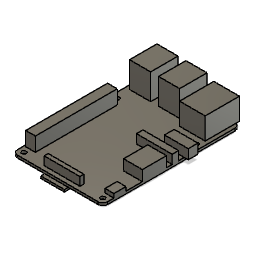
tut_v3.f3d v1 (Autodesk Fusion 360 archive; units mm, degrees)
design "Rough Pi Model"
Autodesk Fusion 360 part; units mm, degrees
sketch "PCB" plane through (0, 0, 0) normal (0, 1, 0) x (1, 0, 0) in component "Raspberry Pi Master"
  line L0 (3, 0) -> (53, 0)
  line L1 (56, -3) -> (56, -82)
  line L2 (53, -85) -> (3, -85)
  line L3 (0, -82) -> (0, -3)
  arc A0 (3, 0) -> (0, -3) centre (3, -3) ccw
  arc A1 (56, -3) -> (53, 0) centre (53, -3) ccw
  arc A2 (53, -85) -> (56, -82) centre (53, -82) ccw
  arc A3 (0, -82) -> (3, -85) centre (3, -82) ccw
  circle A4 centre (52.5, -81.5) radius 1.375
  circle A5 centre (3.5, -81.5) radius 1.375
  circle A6 centre (3.5, -23.5) radius 1.375
  line L4 (3.5, -81.5) -> (3.5, -23.5) construction
  circle A7 centre (52.5, -23.5) radius 1.375
  line L5 (52.5, -23.5) -> (3.5, -23.5) construction
  line L6 (52.5, -23.5) -> (52.5, -81.5) construction
  point P0 (56, 0)
  point P1 (0, -85)
  dimension "d1" = 56
  dimension "d2" = 85
  dimension "d3" = 3
  dimension "d4" = 3
  dimension "d5" = 3
  dimension "d6" = 3
  dimension "d7" = 2.75
  dimension "d8" = 3.5
  dimension "d9" = 3.5
  dimension "d10" = 3.5
  dimension "d11" = 3.5
  dimension "d12" = 58
  constraint horizontal L0
  constraint vertical L1
  constraint horizontal L2
  constraint vertical L3
  constraint coincident origin L3
  constraint coincident origin L0
  constraint tangent L3 A0
  constraint tangent L0 A0
  constraint coincident P0 L0
  constraint coincident P0 L1
  constraint tangent L0 A1
  constraint tangent L1 A1
  constraint tangent L1 A2
  constraint tangent L2 A2
  constraint coincident P1 L2
  constraint coincident P1 L3
  constraint tangent L2 A3
  constraint tangent L3 A3
  constraint equal A4 A5
  constraint coincident A5.centre L4.start
  constraint coincident A6.centre L4.end
  constraint vertical L4
  constraint coincident A7.centre L5.start
  constraint coincident A4.centre L6.end
  constraint vertical L6
  constraint horizontal L5
  constraint equal A4 A7
  constraint equal A4 A6
  measures "d1" distance of origin P0
  measures "d2" distance of origin P1
  measures "d3" radius of A0
  measures "d4" radius of A1
  measures "d5" radius of A2
  measures "d6" radius of A3
  measures "d7" diameter of A4
  measures "d8" distance of L2 A4.centre
  measures "d9" distance of L1 A4.centre
  measures "d10" distance of L2 A5.centre
  measures "d11" distance of L3 A5.centre
  measures "d12" vertical distance of A5.centre A6.centre
extrude "Extrude1" add sketch "PCB" along normal blind 1.5 in component "Raspberry Pi Master"
sketch "Front IO" plane through (0, 1.5, 0) normal (0, 1, 0) x (-1, 0, 0) in component "Raspberry Pi Master"
  circle A0 centre (-52.5, 81.5) radius 1.375
  circle A1 centre (-3.5, 81.5) radius 1.375
  circle A2 centre (-3.5, 23.5) radius 1.375
  circle A3 centre (-52.5, 23.5) radius 1.375
  arc A4 (-3, 0) -> (0, 3) centre (-3, 3) ccw
  line L0 (0, 3) -> (0, 82)
  arc A5 (0, 82) -> (-3, 85) centre (-3, 82) ccw
  line L1 (-3, 85) -> (-53, 85)
  arc A6 (-53, 85) -> (-56, 82) centre (-53, 82) ccw
  line L2 (-56, 82) -> (-56, 3)
  arc A7 (-56, 3) -> (-53, 0) centre (-53, 3) ccw
  line L3 (-53, 0) -> (-3, 0)
  line L4 (-2.45, -2.1) -> (-15.55, -2.1)
  line L5 (-15.55, -2.1) -> (-15.55, 14.9)
  line L6 (-15.55, 14.9) -> (-2.45, 14.9)
  line L7 (-2.45, 14.9) -> (-2.45, -2.1)
  line L8 (-20.45, -2.1) -> (-33.55, -2.1)
  line L9 (-33.55, -2.1) -> (-33.55, 14.9)
  line L10 (-33.55, 14.9) -> (-20.45, 14.9)
  line L11 (-20.45, 14.9) -> (-20.45, -2.1)
  line L12 (-27, -2.1) -> (-56, -2.1) construction
  line L13 (-9, -2.1) -> (-27, -2.1) construction
  line L14 (-56, 3) -> (-56, -2.1) construction
  line L15 (-53.65, -2.1) -> (-37.75, -2.1)
  line L16 (-37.75, -2.1) -> (-37.75, 19.15)
  line L17 (-37.75, 19.15) -> (-53.65, 19.15)
  line L18 (-53.65, 19.15) -> (-53.65, -2.1)
  line L19 (-15.55, 14.9) -> (-20.45, 14.9) construction
  dimension "d15" = 29
  dimension "d16" = 47
  dimension "d17" = 13.1
  dimension "d18" = 2.1
  dimension "d19" = 4.2
  dimension "d21" = 15.9
  dimension "d22" = 21.25
  dimension "d23" = 17
  constraint horizontal L4
  constraint vertical L5
  constraint horizontal L6
  constraint vertical L7
  constraint horizontal L8
  constraint vertical L9
  constraint horizontal L10
  constraint vertical L11
  constraint midpoint L8 L12.start
  constraint parallel L8 L12
  constraint midpoint L4 L13.start
  constraint parallel L4 L13
  constraint coincident L2.end A7.start
  constraint tangent A7 L14
  constraint coincident L12.end L14.end
  constraint equal L6 L10
  constraint horizontal L15
  constraint vertical L16
  constraint horizontal L17
  constraint vertical L18
  constraint coincident L12 L15.start
  constraint horizontal L19
  measures "d15" distance of L12.start L12.end
  measures "d16" distance of L12.end L13.start
  measures "d17" distance of L9.end L10.end
  measures "d18" distance of L3 L12
  measures "d19" distance of L9 L16
  measures "d21" distance of L16.end L17.end
  measures "d22" distance of L15.start L17.end
  measures "d23" distance of L8 L10
extrude "Extrude2" add sketch "Front IO" along normal blind 13.5 contours A7 L3 L15 L16 L18 | A7 L3 L16 L17 L18 in component "Raspberry Pi Master"
extrude "Extrude3" add sketch "Front IO" along normal blind 16 contours A4 L3 L5 L6 L7 | A4 L3 L4 L5 L7 | L3 L8 L9 L11 | L3 L9 L10 L11 in component "Raspberry Pi Master"
sketch "Right IO" plane through (0, 1.5, 0) normal (0, 1, 0) x (-1, 0, 0) in component "Raspberry Pi Master"
  line L0 (-20.45, 14.9) -> (-20.45, 0)
  line L1 (-20.45, 0) -> (-15.55, 0)
  line L2 (-15.55, 0) -> (-15.55, 14.9)
  line L3 (-15.55, 14.9) -> (-2.45, 14.9)
  line L4 (-2.45, 14.9) -> (-2.45, 0.0508)
  arc A0 (-2.45, 0.0508) -> (0, 3) centre (-3, 3) ccw
  line L5 (0, 3) -> (0, 82)
  arc A1 (0, 82) -> (-3, 85) centre (-3, 82) ccw
  line L6 (-3, 85) -> (-53, 85)
  arc A2 (-53, 85) -> (-56, 82) centre (-53, 82) ccw
  line L7 (-56, 82) -> (-56, 3)
  arc A3 (-56, 3) -> (-53.65, 0.0713) centre (-53, 3) ccw
  line L8 (-53.65, 0.0713) -> (-53.65, 19.15)
  line L9 (-53.65, 19.15) -> (-37.75, 19.15)
  line L10 (-37.75, 19.15) -> (-37.75, 0)
  line L11 (-37.75, 0) -> (-33.55, 0)
  line L12 (-33.55, 0) -> (-33.55, 14.9)
  line L13 (-33.55, 14.9) -> (-20.45, 14.9)
  circle A4 centre (-52.5, 81.5) radius 1.375
  circle A5 centre (-3.5, 81.5) radius 1.375
  circle A6 centre (-3.5, 23.5) radius 1.375
  circle A7 centre (-52.5, 23.5) radius 1.375
  line L14 (-50.5, 78.15) -> (-56.1, 78.15)
  line L15 (-56.1, 78.15) -> (-56.1, 70.65)
  line L16 (-56.1, 70.65) -> (-50.5, 70.65)
  line L17 (-50.5, 70.65) -> (-50.5, 78.15)
  line L18 (-44.35, 45.5) -> (-56.1, 45.5)
  line L19 (-56.1, 45.5) -> (-56.1, 60.5)
  line L20 (-56.1, 60.5) -> (-44.35, 60.5)
  line L21 (-44.35, 60.5) -> (-44.35, 45.5)
  line L22 (-56.1, 53) -> (-56.1, 74.4) construction
  line L23 (-56, 42) -> (-33.85, 42)
  line L24 (-33.85, 42) -> (-33.85, 38)
  line L25 (-33.85, 38) -> (-56, 38)
  line L26 (-56, 38) -> (-56, 42)
  line L27 (-58.5, 34.5) -> (-43.75, 34.5)
  line L28 (-43.75, 34.5) -> (-43.75, 28.5)
  line L29 (-43.75, 28.5) -> (-58.5, 28.5)
  line L30 (-58.5, 28.5) -> (-58.5, 34.5)
  point P0 (-56, 40)
  point P1 (-58.5, 31.5)
  dimension "d28" = 10.6
  dimension "d29" = 32
  dimension "d30" = 13
  dimension "d31" = 53.5
  dimension "d32" = 7.5
  dimension "d33" = 15
  dimension "d34" = 4
  dimension "d35" = 6
  dimension "d36" = 58.5
  dimension "d37" = 5.6
  dimension "d38" = 0.1
  dimension "d39" = 11.75
  dimension "d40" = 22.15
  dimension "d41" = 14.75
  constraint horizontal L14
  constraint vertical L15
  constraint horizontal L16
  constraint vertical L17
  constraint horizontal L18
  constraint vertical L19
  constraint horizontal L20
  constraint vertical L21
  constraint midpoint L19 L22.start
  constraint midpoint L15 L22.end
  constraint vertical L22
  constraint horizontal L23
  constraint vertical L24
  constraint horizontal L25
  constraint vertical L26
  constraint coincident L7 L23.start
  constraint midpoint L26 P0
  constraint horizontal L27
  constraint vertical L28
  constraint horizontal L29
  constraint vertical L30
  constraint midpoint L30 P1
  measures "d28" distance of L6 L22.end
  measures "d29" distance of L6 L22.start
  measures "d30" vertical distance of L22.start P0
  measures "d31" distance of L6 P1
  measures "d32" distance of L14.start L16.end
  measures "d33" distance of L18.start L20.end
  measures "d34" distance of L23.end L24.end
  measures "d35" distance of L27.end L28.end
  measures "d36" distance of L5 L30
  measures "d37" distance of L15 L17
  measures "d38" distance of L7 L22
  measures "d39" distance of L19 L21
  measures "d40" distance of L24 L26
  measures "d41" distance of L28 L30
extrude "Extrude4" add sketch "Right IO" along normal blind 6 contours L7 L27 L29 L30 | L7 L27 L28 L29 in component "Raspberry Pi Master"
extrude "Extrude5" add sketch "Right IO" along normal blind 5.5 contours L7 L23 L24 L25 L26 in component "Raspberry Pi Master"
extrude "Extrude6" add sketch "Right IO" along normal blind 6.5 contours L7 L18 L20 L21 in component "Raspberry Pi Master"
extrude "Extrude7" add sketch "Right IO" along normal blind 2.45 contours L7 L14 L16 L17 in component "Raspberry Pi Master"
sketch "SD Card" plane through (0, 0, 0) normal (0, -1, 0) x (1, 0, 0) in component "Raspberry Pi Master"
  circle A0 centre (52.5, 81.5) radius 1.375
  circle A1 centre (3.5, 81.5) radius 1.375
  circle A2 centre (3.5, 23.5) radius 1.375
  circle A3 centre (52.5, 23.5) radius 1.375
  arc A4 (0, 3) -> (3, 0) centre (3, 3) ccw
  line L0 (3, 0) -> (53, 0)
  arc A5 (53, 0) -> (56, 3) centre (53, 3) ccw
  line L1 (56, 3) -> (56, 82)
  arc A6 (56, 82) -> (53, 85) centre (53, 82) ccw
  line L2 (53, 85) -> (3, 85)
  arc A7 (3, 85) -> (0, 82) centre (3, 82) ccw
  line L3 (0, 82) -> (0, 3)
  line L4 (34.5, 87.42) -> (19.9, 87.42)
  line L5 (19.9, 87.42) -> (19.9, 70.4)
  line L6 (19.9, 70.4) -> (34.5, 70.4)
  line L7 (34.5, 70.4) -> (34.5, 87.42)
  dimension "d51" = 19.9
  dimension "d52" = 14.6
  dimension "d53" = 14.6
  dimension "d54" = 2.42
  constraint horizontal L4
  constraint vertical L5
  constraint horizontal L6
  constraint vertical L7
  measures "d51" distance of L3 L5
  measures "d52" distance of L4.start L4.end
  measures "d53" distance of L2 L6
  measures "d54" distance of L2 L4
extrude "Extrude8" add sketch "SD Card" along normal blind 1.35 contours L2 L4 L5 L7 | L2 L5 L6 L7 in component "Raspberry Pi Master"
sketch "Back IO" plane through (0, 1.5, 0) normal (0, 1, 0) x (-1, 0, 0) in component "Raspberry Pi Master"
  arc A0 (3, 85) -> (0, 82) centre (3, 82) ccw
  circle A1 centre (-52.5, 81.5) radius 1.375
  circle A2 centre (-3.5, 81.5) radius 1.375
  circle A3 centre (-3.5, 23.5) radius 1.375
  circle A4 centre (-52.5, 23.5) radius 1.375
  line L0 (-56, 78.15) -> (-50.5, 78.15)
  line L1 (-50.5, 78.15) -> (-50.5, 70.65)
  line L2 (-50.5, 70.65) -> (-56, 70.65)
  line L3 (-56, 70.65) -> (-56, 60.5)
  line L4 (-56, 60.5) -> (-44.35, 60.5)
  line L5 (-44.35, 60.5) -> (-44.35, 45.5)
  line L6 (-44.35, 45.5) -> (-56, 45.5)
  line L7 (-56, 45.5) -> (-56, 42)
  line L8 (-56, 42) -> (-33.85, 42)
  line L9 (-33.85, 42) -> (-33.85, 38)
  line L10 (-33.85, 38) -> (-56, 38)
  line L11 (-56, 38) -> (-56, 34.5)
  line L12 (-56, 34.5) -> (-43.75, 34.5)
  line L13 (-43.75, 34.5) -> (-43.75, 28.5)
  line L14 (-43.75, 28.5) -> (-56, 28.5)
  line L15 (-56, 28.5) -> (-56, 3)
  arc A5 (-56, 3) -> (-53.65, 0.0713) centre (-53, 3) ccw
  line L16 (-53.65, 0.0713) -> (-53.65, 19.15)
  line L17 (-53.65, 19.15) -> (-37.75, 19.15)
  line L18 (-37.75, 19.15) -> (-37.75, 0)
  line L19 (-37.75, 0) -> (-33.55, 0)
  line L20 (-33.55, 0) -> (-33.55, 14.9)
  line L21 (-33.55, 14.9) -> (-20.45, 14.9)
  line L22 (-20.45, 14.9) -> (-20.45, 0)
  line L23 (-20.45, 0) -> (-15.55, 0)
  line L24 (-15.55, 0) -> (-15.55, 14.9)
  line L25 (-15.55, 14.9) -> (-2.45, 14.9)
  line L26 (-2.45, 14.9) -> (-2.45, 0.0508)
  arc A6 (-2.45, 0.0508) -> (0, 3) centre (-3, 3) ccw
  line L27 (0, 3) -> (0, 82)
  arc A7 (0, 82) -> (-3, 85) centre (-3, 82) ccw
  line L28 (-3, 85) -> (-53, 85)
  arc A8 (-53, 85) -> (-56, 82) centre (-53, 82) ccw
  line L29 (-56, 82) -> (-56, 78.15)
  line L30 (-16.9, 79.85) -> (-39.1, 79.85)
  line L31 (-39.1, 79.85) -> (-39.1, 82.35)
  line L32 (-39.1, 82.35) -> (-16.9, 82.35)
  line L33 (-16.9, 82.35) -> (-16.9, 79.85)
  dimension "d57" = 28
  dimension "d58" = 2.5
  dimension "d59" = 2.65
  dimension "d60" = 22.2
  constraint horizontal L30
  constraint vertical L31
  constraint horizontal L32
  constraint vertical L33
  measures "d58" distance of L30.end L31.end
  measures "d59" distance of L28 L31.end
  measures "d60" distance of L30.start L30.end
extrude "Extrude9" add sketch "Back IO" along normal blind 5.25 contours L30 L31 L32 L33 in component "Raspberry Pi Master"
sketch "GPIO" plane through (0, 1.5, 0) normal (0, 1, 0) x (-1, 0, 0) in component "Raspberry Pi Master"
  arc A0 (-53, 85) -> (-56, 82) centre (-53, 82) ccw
  line L0 (-16.9, 82.35) -> (-16.9, 79.85)
  line L1 (-16.9, 79.85) -> (-39.1, 79.85)
  line L2 (-39.1, 79.85) -> (-39.1, 82.35)
  line L3 (-39.1, 82.35) -> (-16.9, 82.35)
  circle A1 centre (-52.5, 81.5) radius 1.375
  circle A2 centre (-3.5, 81.5) radius 1.375
  circle A3 centre (-3.5, 23.5) radius 1.375
  circle A4 centre (-52.5, 23.5) radius 1.375
  line L4 (-56, 78.15) -> (-50.5, 78.15)
  line L5 (-50.5, 78.15) -> (-50.5, 70.65)
  line L6 (-50.5, 70.65) -> (-56, 70.65)
  line L7 (-56, 70.65) -> (-56, 60.5)
  line L8 (-56, 60.5) -> (-44.35, 60.5)
  line L9 (-44.35, 60.5) -> (-44.35, 45.5)
  line L10 (-44.35, 45.5) -> (-56, 45.5)
  line L11 (-56, 45.5) -> (-56, 42)
  line L12 (-56, 42) -> (-33.85, 42)
  line L13 (-33.85, 42) -> (-33.85, 38)
  line L14 (-33.85, 38) -> (-56, 38)
  line L15 (-56, 38) -> (-56, 34.5)
  line L16 (-56, 34.5) -> (-43.75, 34.5)
  line L17 (-43.75, 34.5) -> (-43.75, 28.5)
  line L18 (-43.75, 28.5) -> (-56, 28.5)
  line L19 (-56, 28.5) -> (-56, 3)
  arc A5 (-56, 3) -> (-53.65, 0.0713) centre (-53, 3) ccw
  line L20 (-53.65, 0.0713) -> (-53.65, 19.15)
  line L21 (-53.65, 19.15) -> (-37.75, 19.15)
  line L22 (-37.75, 19.15) -> (-37.75, 0)
  line L23 (-37.75, 0) -> (-33.55, 0)
  line L24 (-33.55, 0) -> (-33.55, 14.9)
  line L25 (-33.55, 14.9) -> (-20.45, 14.9)
  line L26 (-20.45, 14.9) -> (-20.45, 0)
  line L27 (-20.45, 0) -> (-15.55, 0)
  line L28 (-15.55, 0) -> (-15.55, 14.9)
  line L29 (-15.55, 14.9) -> (-2.45, 14.9)
  line L30 (-2.45, 14.9) -> (-2.45, 0.0508)
  arc A6 (-2.45, 0.0508) -> (0, 3) centre (-3, 3) ccw
  line L31 (0, 3) -> (0, 82)
  arc A7 (0, 82) -> (-3, 85) centre (-3, 82) ccw
  line L32 (-3, 85) -> (-53, 85)
  arc A8 (-53, 85) -> (-56, 82) centre (-53, 82) ccw
  line L33 (-56, 82) -> (-56, 78.15)
  line L34 (-1, 27.1) -> (-7, 27.1)
  line L35 (-7, 27.1) -> (-7, 77.9)
  line L36 (-7, 77.9) -> (-1, 77.9)
  line L37 (-1, 77.9) -> (-1, 27.1)
  circle A9 centre (-3.5, 81.5) radius 1.375
  dimension "d63" = 29
  dimension "d64" = 50.8
  dimension "d65" = 1
  dimension "d66" = 6
  constraint horizontal L34
  constraint vertical L35
  constraint horizontal L36
  constraint vertical L37
  measures "d64" distance of L34 L36
  measures "d65" distance of L31 L37
  measures "d66" distance of L35.end L36.end
extrude "Extrude10" add sketch "GPIO" along normal blind 8.75 contours L34 L35 L36 L37 in component "Raspberry Pi Master"
component "Raspberry Pi Master" placed x (1, 0, 0) y (0, 1, 0) z (0, 0, 1) at (0, 0, 0)
